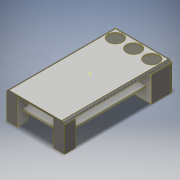
# Autodesk Inventor part: TABLE
Saved by Autodesk Inventor 2019 (Build 230136000, 136)
## iProperties
Created: 2018-12-01
Part Number: TABLE
Material: Generic
Document SubType Name: Modeling
Designer: Manoj
Density: 1 g/cm^3
Appearance: Silver
Author: Manoj
Autodesk Inventor part; units mm, degrees
ref_plane "YZ Plane" through (0, 0, 0) normal (1, 0, 0) x (0, 1, 0)
ref_plane "XY Plane" through (0, 0, 0) normal (0, 0, 1) x (1, 0, 0)
sketch "Sketch1" plane through (0, 0, 0) normal (0, 1, 0) x (-1, 0, 0)
  line L0 (400, 750) -> (-400, 750)
  line L1 (-400, 750) -> (-400, -750)
  line L2 (-400, -750) -> (400, -750)
  line L3 (400, -750) -> (400, 750)
  point P0 (0, 0)
  dimension "d0" = 1500
  dimension "d1" = 800
  dimension "d2" = 400
  dimension "d3" = 750
  constraints: 8 end point, 2 parallel, 1 horizontal, 1 perpendicular
  measures "d0" distance of L2.end L0.start
  measures "d1" distance of L0.start L0.end
  measures "d2" distance from line of point (0, 0) L3
  measures "d3" distance from line of L0 point (0, 0)
sketch "Sketch2" plane through (0, 0, 0) normal (0, 1, 0) x (-1, 0, 0)
  line L0 (400, -750) -> (400, 750) projected
  line L1 (400, 750) -> (-400, 750) projected
  line L2 (-400, -750) -> (400, -750) projected
  line L3 (-400, 750) -> (-400, -750) projected
  line L4 (400, 750) -> (400, 600)
  line L5 (400, 600) -> (250, 600)
  line L6 (250, 600) -> (250, 750)
  line L7 (-400, 750) -> (-250, 750)
  line L8 (-250, 750) -> (-250, 600)
  line L9 (-250, 600) -> (-400, 600)
  line L10 (400, 0) -> (-400, 0) construction
  line L11 (400, -600) -> (250, -600)
  line L12 (250, -600) -> (250, -750)
  line L13 (-250, -750) -> (-250, -600)
  line L14 (-250, -600) -> (-400, -600)
  line L15 (250, -750) -> (400, -750)
  line L16 (400, -600) -> (400, -750)
  line L17 (-400, -750) -> (-250, -750)
  line L18 (-400, -750) -> (-400, -600)
  point P0 (0, 0)
  dimension "d4" = 150
  dimension "d5" = 150
  dimension "d6" = 150
  dimension "d7" = 150
  dimension "d8" = 150
  dimension "d9" = 150
  constraints: 30 end point, 6 symmetric about line, 4 collinear, 4 point on line, 2 midpoint, 2 perpendicular
  measures "d4" distance of L0.end L4.end
  measures "d5" distance of L4.end L5.end
  measures "d6" distance of L5.end L6.end
  measures "d7" distance of L1.end L7.end
  measures "d8" distance of L7.end L8.end
  measures "d9" distance of L8.end L9.end
extrude "Extrusion1" add sketch "Sketch2" against normal blind 360 contours L5 L6 L1 L0
extrude "Extrusion2" add sketch "Sketch2" against normal blind 360 contours L2 L12 L11 L0 | L2 L3 L14 L13 | L8 L9 L3 L1
extrude "Extrusion3" add sketch "Sketch1" along normal blind 25
ref_plane "Work Plane1" through (0, -200, 0) normal (0, 1, 0) x (-1, 0, 0)
sketch "Sketch3" plane through (0, -200, 0) normal (0, 1, 0) x (-1, 0, 0)
  line L0 (250, -750) -> (250, -600) construction
  line L1 (250, -675) -> (325, -675) construction
  line L2 (0, -801.814) -> (0, 857.0329) construction
  line L3 (642.7867, 0) -> (-967.9312, 0) construction
  line L4 (-250, -750) -> (-250, -600) construction
  line L5 (-250, -675) -> (-325, -675) construction
  line L6 (250, 675) -> (325, 675) construction
  line L7 (-250, 675) -> (-325, 675) construction
  line L8 (325, -675) -> (-325, -675)
  line L9 (-325, -675) -> (-325, 675)
  line L10 (-325, 675) -> (325, 675)
  line L11 (325, 675) -> (325, -675)
  point P0 (0, 0)
  dimension "d17" = 75
  constraints: 22 end point, 8 symmetric about line, 3 horizontal, 2 parallel, 1 midpoint, 1 perpendicular, 1 vertical
  measures "d17" distance of L1.start L1.end
extrude "Extrusion4" add sketch "Sketch3" along normal blind 25
sketch "Sketch4" plane through (-250, -360, -600) normal (1, 0, 0) x (0, 0, -1)
  line L0 (150, 385) -> (-1350, 385) projected
  line L1 (0, 0) -> (150, 0) projected
  line L2 (116.9952, 385) -> (150, 385)
  line L3 (150, 385) -> (150, 0)
  line L4 (150, 0) -> (116.9952, 0)
  line L5 (116.9952, 0) -> (116.9952, 385)
  point P0 (-600, 360)
  constraints: 8 end point, 2 parallel, 1 horizontal, 1 perpendicular, 1 point on line
extrude "Extrusion5" add sketch "Sketch4" along normal blind 588.75
sketch "Sketch5" plane through (-250, -360, 750) normal (1, 0, 0) x (0, 0, -1)
  point P0 (750, 360)
sketch "Sketch6" plane through (-250, -175, -600) normal (1, 0, 0) x (0, 0, -1)
  line L0 (0, 175) -> (-1200, 175) projected
  line L1 (0, -185) -> (150, -185) projected
  line L2 (0, 175) -> (112.5772, 175)
  line L3 (112.5772, 175) -> (112.5772, -185)
  line L4 (112.5772, -185) -> (0, -185)
  line L5 (0, -185) -> (0, 175)
  point P0 (-600, 175)
  constraints: 8 end point, 2 parallel, 1 horizontal, 1 perpendicular, 1 point on line
extrude "Extrusion6" add sketch "Sketch6" along normal blind 588.75
sketch "Sketch7" plane through (-400, -360, -600) normal (0, 0, 1) x (1, 0, 0)
  line L0 (800, 360) -> (800, 0) projected
  line L1 (0, 385) -> (800, 385)
  line L2 (800, 385) -> (800, 0)
  line L3 (800, 0) -> (0, 0)
  line L4 (0, 0) -> (0, 385)
  point P0 (400, 360)
  constraints: 8 end point, 2 parallel, 1 horizontal, 1 perpendicular
extrude "Extrusion7" add sketch "Sketch7" along normal blind 155.25
sketch "Sketch8" plane through (0, 0, 0) normal (1, 0, 0) x (0, 1, 0)
  line L0 (0, -462.2615) -> (-345.7489, -462.2615)
  line L1 (-345.7489, -462.2615) -> (-345.7489, -736.9661)
  line L2 (-345.7489, -736.9661) -> (0, -736.9661)
  line L3 (0, -736.9661) -> (0, -462.2615)
  point P0 (0, 0)
  constraints: 8 end point, 2 parallel, 1 horizontal, 1 perpendicular
extrude "Extrusion8" cut sketch "Sketch8" along normal mid plane 790
sketch "Sketch9" plane through (0, 25, 0) normal (0, 1, 0) x (1, 0, 0)
  line L0 (400, -750) -> (400, 750) construction
  point P0 (0, 0)
sketch "Sketch10" plane through (0, 25, 0) normal (0, 1, 0) x (1, 0, 0)
  line L0 (400, -750) -> (400, 750) construction
  line L1 (400, 750) -> (250, 750) construction
  line L2 (400, 600) -> (400, 750) construction
  circle A0 centre (250, 600) radius 100
  point P0 (0, 0)
  dimension "d33" = 200
  constraints: 4 end point, 1 centre point, 1 horizontal
  measures "d33" diameter of A0
extrude "Extrusion9" cut sketch "Sketch10" against normal blind 10
pattern_linear "Rectangular Pattern1" count 3 spacing 250 along (-1, 0, 0) of "Extrusion9"
sketch "Sketch12" plane through (-400, -360, -444.75) normal (0, 0, 1) x (1, 0, 0)
  line L0 (650, 360) -> (650, 0) projected
  line L1 (568.3872, 318.9469) -> (650, 318.9469)
  line L2 (650, 318.9469) -> (650, 241.0156)
  line L3 (650, 241.0156) -> (568.3872, 241.0156)
  line L4 (568.3872, 241.0156) -> (568.3872, 318.9469)
  point P0 (400, 360)
  constraints: 8 end point, 2 parallel, 1 horizontal, 1 perpendicular, 1 point on line
extrude "Extrusion10" add sketch "Sketch12" along normal blind 10
sketch "Sketch13" plane through (-400, -360, -434.75) normal (0, 0, 1) x (1, 0, 0)
  line L0 (596.3872, 318.0662) -> (621.3872, 318.0662)
  line L1 (621.3872, 318.0662) -> (621.3872, 292.1316)
  line L2 (621.3872, 292.1316) -> (596.3872, 292.1316)
  line L3 (596.3872, 292.1316) -> (596.3872, 318.0662)
  line L4 (646.3872, 282.3185) -> (621.3872, 282.3185)
  line L5 (621.3872, 282.3185) -> (621.3872, 259.4213)
  line L6 (621.3872, 259.4213) -> (646.3872, 259.4213)
  line L7 (646.3872, 259.4213) -> (646.3872, 282.3185)
  line L8 (596.3872, 282.3185) -> (571.3872, 282.3185)
  line L9 (571.3872, 282.3185) -> (571.3872, 259.4213)
  line L10 (571.3872, 259.4213) -> (596.3872, 259.4213)
  line L11 (596.3872, 259.4213) -> (596.3872, 282.3185)
  line L12 (568.3872, 318.9469) -> (568.3872, 241.0156) projected
  point P0 (400, 360)
  dimension "d41" = 25
  dimension "d42" = 25
  dimension "d43" = 25
  dimension "d44" = 3
  constraints: 24 end point, 6 parallel, 3 horizontal, 3 perpendicular, 3 point on line, 1 collinear
  measures "d41" distance of L8.start L8.end
  measures "d42" distance of L4.start L4.end
  measures "d43" distance of L1.end L2.end
  measures "d44" distance between parallel lines of L12 L9
extrude "Extrusion11" cut sketch "Sketch13" against normal blind 30
fillet "Fillet1" radius 40 1 edges at (0, 25, -750)
fillet "Fillet2" radius 40 6 edges at (-400, 13.2843, -738.2843) (-400, 25, 20) (-400, -187.5, -750) (400, 13.2843, -738.2843) (400, 25, 20) (400, -187.5, -750)
body "Solid1"
